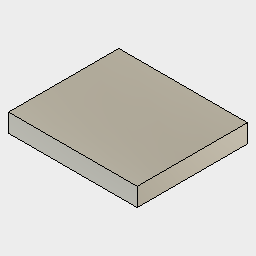
bottom (Autodesk Fusion 360 design; units mm, degrees)
Autodesk Fusion 360 part; units mm, degrees
note: some values were not read from the file. Chosen so that the rebuilt part matches the saved one: which face or edge a step refers to.
box "BoxPrimitive1" add length 50.8 width 95.25 height 1.5875 placed x (0, 1, 0) y (-1, 0, 0) z (0, 0, 1) at (95.25, 0, 0) makes body 1 in component "Battery Plate"
sketch "Sketch2" plane through (0, 0, 1.5875) normal (0, 0, 1) x (-1, 0, 0) in component "Battery Plate"
  line L0 (-95.25, -50.8) -> (0, -50.8)
  line L1 (0, -50.8) -> (0, 0)
  line L2 (0, 0) -> (-95.25, 0)
  line L3 (-95.25, 0) -> (-95.25, -50.8)
  circle A0 centre (-86.995, -25.4) radius 2.413
  circle A1 centre (-8.255, -25.4) radius 2.413
  point P0 (-47.625, -25.4)
  point P1 (-8.255, -25.4)
  point P2 (-86.995, -25.4)
  dimension "d49" = 4.826
  dimension "d50" = 4.826
  measures "d49" diameter of A0
  measures "d50" diameter of A1
extrude "Extrude1" cut sketch "Sketch2" against normal blind 1.5875 contours A0 | A1 bodies 1 in component "Battery Plate"
fillet "Fillet1" radius 1.27 4 edges at (47.625, 0, 1.5875) (0, 25.4, 1.5875) (47.625, 50.8, 1.5875) (95.25, 25.4, 1.5875) on bodies 1 in component "Battery Plate"
fillet "Fillet2" radius 1.27 8 edges at (95.25, 0, 0.1588) (94.878, 0.372, 1.2155) (0, 0, 0.1588) (0.372, 0.372, 1.2155) (94.878, 50.428, 1.2155) (95.25, 50.8, 0.1588) (0, 50.8, 0.1588) (0.372, 50.428, 1.2155) on bodies 1 in component "Battery Plate"
box "BoxPrimitive1'" add length 114.3 width 133.35 height 19.05 placed x (0, 1, 0) y (-1, 0, 0) z (0, 0, 1) at (133.35, 0, 0) separate body makes body 2 in component "Fillet"
fillet "Fillet1'" radius 12.7 2 edges at (66.675, 0, 19.05) (66.675, 114.3, 19.05) on bodies 2 in component "Fillet"
box "BoxPrimitive1''" add length 114.3 width 133.35 height 19.05 placed x (0, 1, 0) y (-1, 0, 0) z (0, 0, 1) at (133.35, 0, 0) separate body makes body 3 in component "Inside"
sketch "Sketch2 (2)" plane through (0, 0, 19.05) normal (0, 0, 1) x (-1, 0, 0) in component "Inside"
  line L0 (-133.35, -114.3) -> (0, -114.3)
  line L1 (0, -114.3) -> (0, 0)
  line L2 (0, 0) -> (-133.35, 0)
  line L3 (-133.35, 0) -> (-133.35, -114.3)
  line L4 (0, -3.302) -> (-133.35, -3.302)
  line L5 (-133.35, -3.302) -> (-133.35, -9.779)
  line L6 (0, -9.779) -> (0, -3.302)
  line L7 (0, -110.998) -> (-133.35, -110.998)
  line L8 (-133.35, -110.998) -> (-133.35, -107.696)
  line L9 (0, -107.696) -> (0, -110.998)
  line L10 (-32.385, -85.09) -> (-100.965, -85.09)
  line L11 (-100.965, -85.09) -> (-100.965, -29.21)
  line L12 (-100.965, -29.21) -> (-32.385, -29.21)
  line L13 (-32.385, -29.21) -> (-32.385, -85.09)
  line L14 (-9.525, -107.696) -> (-9.525, -9.779)
  line L15 (-123.825, -107.696) -> (-123.825, -9.779)
  line L16 (-133.35, -107.696) -> (-123.825, -107.696)
  line L17 (-9.525, -107.696) -> (0, -107.696)
  line L18 (-133.35, -9.779) -> (-123.825, -9.779)
  line L19 (-9.525, -9.779) -> (0, -9.779)
  circle A0 centre (-106.045, -57.15) radius 1.6002
  circle A1 centre (-27.305, -57.15) radius 1.6002
  point P0 (0, -3.302)
  point P1 (0, -110.998)
  point P2 (-133.35, -107.696)
  point P3 (-32.385, -85.09)
  point P4 (-100.965, -29.21)
  point P5 (-106.045, -57.15)
  point P6 (-27.305, -57.15)
  dimension "d141" = 3.2004
  dimension "d142" = 3.2004
  measures "d141" diameter of A0
  measures "d142" diameter of A1
extrude "Extrude1'" cut sketch "Sketch2 (2)" against normal blind 6.35 contours L1 L3 L4 L5 L6 L7 L8 L9 L14 L15 L16 L17 L18 L19 bodies 3 in component "Inside"
extrude "Extrude2" cut sketch "Sketch2 (2)" against normal blind 15.24 contours L10 L11 L12 L13 bodies 3 in component "Inside"
extrude "Extrude3" cut sketch "Sketch2 (2)" against normal blind 13.97 contours A0 | A1 bodies 3 in component "Inside"
box "BoxPrimitive1'''" add length 114.3 width 133.35 height 20.32 placed x (0, 1, 0) y (-1, 0, 0) z (0, 0, 1) at (133.35, 0, 0) separate body makes body 4 in component "Face"
box "BoxPrimitive2" add length 114.3 width 133.35 height 19.05 placed x (0, 1, 0) y (-1, 0, 0) z (0, 0, 1) at (133.35, 0, 0) separate body makes body 5 in component "Face"
extrude "Extrude1''" add 1 faces at (88.9, 38.1, 20.32) along direction (0, 0, 1) blind 0.508 on bodies 4 bodies 4 in component "Face"
component "Battery Plate" placed x (1, 0, 0) y (0, 1, 0) z (0, 0, 1) at (0, 0, 0)
component "Fillet" placed x (1, 0, 0) y (0, 1, 0) z (0, 0, 1) at (0, 0, 0)
component "Inside" placed x (1, 0, 0) y (0, 1, 0) z (0, 0, 1) at (0, 0, 0)
component "Face" placed x (1, 0, 0) y (0, 1, 0) z (0, 0, 1) at (0, 0, 0)
hidden bodies 4
